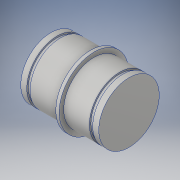
# Autodesk Inventor part: Idle Pivot
Saved by Autodesk Inventor 2019.4 (Build 234330000, 330)
## iProperties
Created: 2020-01-12
Part Number: Idle Pivot
Material: Aluminum 6061
Document SubType Name: Modeling
Designer: admin
Density: 2.7 g/cm^3
Appearance: Aluminum - Flat
Author: admin
Autodesk Inventor part; units mm, degrees
ref_plane "YZ Plane" through (0, 0, 0) normal (1, 0, 0) x (0, 1, 0)
ref_plane "XZ Plane" through (0, 0, 0) normal (0, 1, 0) x (-1, 0, 0)
ref_plane "XY Plane" through (0, 0, 0) normal (0, 0, 1) x (1, 0, 0)
sketch "Sketch1" plane through (0, 0, 0) normal (0, 0, 1) x (1, 0, 0)
  line L0 (0, 0) -> (0, 10)
  line L1 (13.1, 10) -> (13.1, 11.5)
  line L2 (13.1, 11.5) -> (14.2, 11.5)
  line L3 (14.2, 11.5) -> (14.2, 10)
  line L4 (14.2, 10) -> (22.7, 10)
  line L5 (22.7, 10) -> (22.7, 9.5)
  line L6 (22.7, 9.5) -> (23.8, 9.5)
  line L7 (23.8, 9.5) -> (23.8, 10)
  line L8 (23.8, 10) -> (25.8, 10)
  line L9 (25.8, 10) -> (25.8, 0)
  line L10 (25.8, 0) -> (0, 0)
  line L11 (0, 10) -> (2, 10)
  line L12 (2, 10) -> (2, 9.5)
  line L13 (2, 9.5) -> (3.1, 9.5)
  line L14 (3.1, 9.5) -> (3.1, 10)
  line L15 (3.1, 10) -> (13.1, 10)
  dimension "d0" = 2
  dimension "d1" = 1.1
  dimension "d2" = 0.5
  dimension "d3" = 10
  dimension "d4" = 1.1
  dimension "d5" = 0.5
  dimension "d6" = 8.5
  dimension "d7" = 1.1
  dimension "d8" = 1.5
  dimension "d9" = 10
  dimension "d10" = 2
  constraints: 32 end point, 12 perpendicular, 3 point on line, 1 collinear, 1 horizontal, 1 vertical
  measures "d0" distance of L0.end L11.end
  measures "d1" distance of L12.end L13.end
  measures "d2" distance of L13.end L14.end
  measures "d3" distance of L14.end L1.start
  measures "d4" distance of L5.end L6.end
  measures "d5" distance of L6.end L7.end
  measures "d6" distance of L3.end L4.end
  measures "d7" distance of L1.end L2.end
  measures "d8" distance of L1.start L1.end
  measures "d9" distance between parallel lines of L10 L15
  measures "d10" distance of L7.end L8.end
revolve "Revolution1" add sketch "Sketch1" angle 360 about axis through (25.8, 0, 0) along (-1, 0, 0)
body "Solid1"
